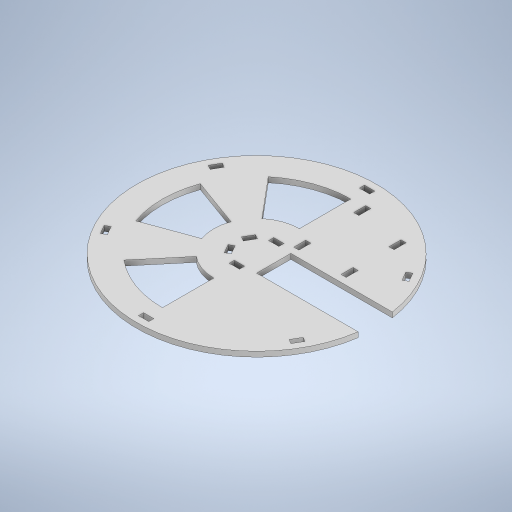
# Autodesk Inventor part: rolling_plate_top
Saved by Autodesk Inventor 2024 (Build 280153000, 153)
## iProperties
Created: 2024-04-09
Part Number: rolling_plate_top
Material: 一般
Document SubType Name: Modeling
Designer: USER
Density: 1 g/cm^3
Appearance: 預設
Author: USER
Autodesk Inventor part; units mm, degrees
ref_plane "YZ Plane" through (0, 0, 0) normal (1, 0, 0) x (0, 1, 0)
ref_plane "XZ Plane" through (0, 0, 0) normal (0, 1, 0) x (-1, 0, 0)
ref_plane "XY Plane" through (0, 0, 0) normal (0, 0, 1) x (1, 0, 0)
sketch "草圖1" plane through (0, 0, 0) normal (0, 1, 0) x (-1, 0, 0)
  circle A0 centre (0, 0) radius 70
  circle A1 centre (0, 0) radius 25
  line L0 (-70, 10) -> (-10, 10)
  line L1 (-10, 10) -> (-10, -10)
  line L2 (-10, -10) -> (-70, -10)
  line L3 (-70, -10) -> (-70, 10)
  line L4 (0, 0) -> (0, -55)
  line L5 (0, 0) -> (35.3533, -42.1324)
  arc A2 (0, -55) -> (35.3533, -42.1324) centre (0, 0) ccw
  line L6 (0, 0) -> (51.6831, -18.8111)
  line L7 (0, 0) -> (51.6831, 18.8111)
  arc A3 (51.6831, -18.8111) -> (51.6831, 18.8111) centre (0, 0) ccw
  line L8 (0, 0) -> (35.3533, 42.1324)
  line L9 (0, 0) -> (0, 55)
  arc A4 (35.3533, 42.1324) -> (0, 55) centre (0, 0) ccw
  line L10 (-9.2, -7) -> (-36.8, -7)
  line L11 (-36.8, -7) -> (-36.8, -63)
  line L12 (-36.8, -63) -> (-9.2, -63)
  line L13 (-9.2, -63) -> (-9.2, -7)
  line L14 (-7.7, -14) -> (-10.7, -14)
  line L15 (-10.7, -14) -> (-10.7, -21)
  line L16 (-10.7, -21) -> (-7.7, -21)
  line L17 (-7.7, -21) -> (-7.7, -14)
  line L18 (-7.7, -49) -> (-10.7, -49)
  line L19 (-10.7, -49) -> (-10.7, -56)
  line L20 (-10.7, -56) -> (-7.7, -56)
  line L21 (-7.7, -56) -> (-7.7, -49)
  line L22 (-35.3, -14) -> (-38.3, -14)
  line L23 (-38.3, -14) -> (-38.3, -21)
  line L24 (-38.3, -21) -> (-35.3, -21)
  line L25 (-35.3, -21) -> (-35.3, -14)
  line L26 (-35.3, -42) -> (-38.3, -42)
  line L27 (-38.3, -42) -> (-38.3, -49)
  line L28 (-38.3, -49) -> (-35.3, -49)
  line L29 (-35.3, -49) -> (-35.3, -42)
  circle A5 centre (0, 0) radius 2
  line L30 (-1.5, 1.3229) -> (-1.5, -1.3229)
  point P0 (-23, -10)
  point P1 (-9.2, -14)
  point P2 (-9.2, -56)
  point P3 (-36.8, -14)
  point P4 (-36.8, -42)
  point P5 (16.0697, -19.1511)
  point P6 (0, -25)
  point P7 (-69.282, 10)
  point P8 (-69.282, -10)
  point P9 (16.0697, 19.1511)
  point P10 (0, 25)
  point P11 (23.4923, -8.5505)
  point P12 (23.4923, 8.5505)
  point P13 (-70, 0)
  point P14 (-10, 0)
  point P15 (-23, -7)
  dimension "d0" = 140
  dimension "d1" = 50
  dimension "d2" = 20
  dimension "d3" = 60
  dimension "d4" = 55
  dimension "d5" = 40
  dimension "d6" = 55
  dimension "d9" = 140
  dimension "d12" = 27.6
  dimension "d13" = 56
  dimension "d14" = 7
  dimension "d15" = 3
  dimension "d16" = 7
  dimension "d17" = 7
  dimension "d18" = 3
  dimension "d19" = 7
  dimension "d20" = 7
  dimension "d21" = 3
  dimension "d22" = 7
  dimension "d23" = 7
  dimension "d24" = 3
  dimension "d25" = 21
  dimension "d28" = 4
  dimension "d29" = 1.5
  dimension "d30" = 17
  dimension "d31" = 17
  dimension "d32" = 13
  constraints: 62 end point, 12 parallel, 8 point on circle, 7 midpoint, 7 point on line, 6 coincident, 6 perpendicular, 5 centre point, 5 horizontal, 2 vertical, 1 horizontal alignment, 1 vertical alignment, 20 other
  measures "d1" diameter of A1
  measures "d2" distance of L2.end L0.start
  measures "d3" distance of L1.end L2.end
  measures "d4" distance of L4.start L4.end
  measures "d5" angle of L4 L5
  measures "d6" distance of L4.start L5.end
  measures "d12" distance of L11.end L12.end
  measures "d13" distance of L12.end L10.start
  measures "d14" distance of L16.end L14.start
  measures "d15" distance of L15.end L16.end
  measures "d16" distance from line of L10.start L14
  measures "d17" distance of L20.end L18.start
  measures "d18" distance of L19.end L20.end
  measures "d19" distance from line of L12.end L20
  measures "d20" distance of L24.end L22.start
  measures "d21" distance of L23.end L24.end
  measures "d22" vertical distance of L10.end L22.start
  measures "d23" distance of L28.end L26.start
  measures "d24" distance of L27.end L28.end
  measures "d25" distance of L24.end L26.start
  measures "d28" diameter of A5
  measures "d29" distance between parallel lines of L4 L30
  measures "d30" distance from line of L0 L10.start
  measures "d31" distance from line of L0 L10.end
  measures "d32" horizontal distance of point (-10, 0) point (-23, -7)
extrude "擠出1" add sketch "草圖1" along normal blind 3 contours A0 L12 L13 L20 L21 L18 A1 L4 A2 L5 L6 A3 L7 L8 A4 L9 L0 | A0 L11 L28 L29 L26 L24 L25 L22 L2 A1 L13 L18 L19 L20 L12 | A1 L9 A5 L4 L13 L16 L17 L14 L10 L1 L0 | A0 L2 L11 L22 L23 L24 L26 L27 L28 | A1 L8 A5 L9 | A1 L7 A5 L8 | A5 L8 L9 | L9 L4 A5 L30 | L2 L1 L10 L13 L14 L15 L16 A1 | A1 L6 A5 L7 | A5 L7 L8 | L5 A5 L4 | L6 A5 L5 | L7 A5 L6 | L30 A5 | A5 L5 A1 L4 | A5 L6 A1 L5
sketch "草圖2" plane through (0, 3, 0) normal (0, 1, 0) x (1, 0, 0)
  line L0 (-3, 13) -> (3, 13)
  line L1 (3, 13) -> (3, 10)
  line L2 (3, 10) -> (-3, 10)
  line L3 (-3, 10) -> (-3, 13)
  line L4 (-12.7583, 3.9019) -> (-9.7583, 9.0981)
  line L5 (-9.7583, 9.0981) -> (-7.1603, 7.5981)
  line L6 (-7.1603, 7.5981) -> (-10.1603, 2.4019)
  line L7 (-10.1603, 2.4019) -> (-12.7583, 3.9019)
  line L8 (-9.7583, -9.0981) -> (-12.7583, -3.9019)
  line L9 (-12.7583, -3.9019) -> (-10.1603, -2.4019)
  line L10 (-10.1603, -2.4019) -> (-7.1603, -7.5981)
  line L11 (-7.1603, -7.5981) -> (-9.7583, -9.0981)
  line L12 (3, -13) -> (-3, -13)
  line L13 (-3, -13) -> (-3, -10)
  line L14 (-3, -10) -> (3, -10)
  line L15 (3, -10) -> (3, -13)
  line L16 (-3, 66) -> (3, 66)
  line L17 (3, 66) -> (3, 63)
  line L18 (3, 63) -> (-3, 63)
  line L19 (-3, 63) -> (-3, 66)
  line L20 (-53.0596, 34.0981) -> (-56.0596, 28.9019)
  line L21 (-56.0596, 28.9019) -> (-58.6577, 30.4019)
  line L22 (-58.6577, 30.4019) -> (-55.6577, 35.5981)
  line L23 (-55.6577, 35.5981) -> (-53.0596, 34.0981)
  line L24 (-56.0596, -28.9019) -> (-53.0596, -34.0981)
  line L25 (-53.0596, -34.0981) -> (-55.6577, -35.5981)
  line L26 (-55.6577, -35.5981) -> (-58.6577, -30.4019)
  line L27 (-58.6577, -30.4019) -> (-56.0596, -28.9019)
  line L28 (-3, -63) -> (3, -63)
  line L29 (3, -63) -> (3, -66)
  line L30 (3, -66) -> (-3, -66)
  line L31 (-3, -66) -> (-3, -63)
  line L32 (53.0596, -34.0981) -> (56.0596, -28.9019)
  line L33 (56.0596, -28.9019) -> (58.6577, -30.4019)
  line L34 (58.6577, -30.4019) -> (55.6577, -35.5981)
  line L35 (55.6577, -35.5981) -> (53.0596, -34.0981)
  line L36 (56.0596, 28.9019) -> (53.0596, 34.0981)
  line L37 (53.0596, 34.0981) -> (55.6577, 35.5981)
  line L38 (55.6577, 35.5981) -> (58.6577, 30.4019)
  line L39 (58.6577, 30.4019) -> (56.0596, 28.9019)
  point P0 (0, 0)
  point P1 (0, 10)
  point P2 (-8.6603, 5)
  point P3 (-8.6603, -5)
  point P4 (0, -10)
  point P5 (0, 63)
  point P6 (-54.5596, 31.5)
  point P7 (-54.5596, -31.5)
  point P8 (0, -63)
  point P9 (54.5596, -31.5)
  point P10 (54.5596, 31.5)
  dimension "d33" = 3
  dimension "d34" = 6
  dimension "d35" = 10
  dimension "d38" = 180
  dimension "d40" = 3
  dimension "d41" = 6
  dimension "d42" = 63
  dimension "d45" = 360
  constraints: 80 end point, 4 parallel, 2 horizontal, 2 midpoint, 2 perpendicular, 2 vertical alignment, 83 other
  measures "d33" distance of L0.end L1.end
  measures "d34" distance of L1.end L2.end
  measures "d35" distance from line of point (0, 0) L2
  measures "d40" distance of L16.end L17.end
  measures "d41" distance of L17.end L18.end
  measures "d42" distance from line of point (0, 0) L18
extrude "擠出2" cut sketch "草圖2" against normal through all
